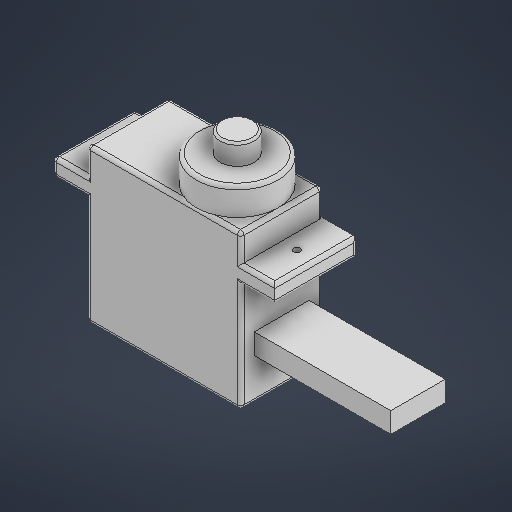
# Autodesk Inventor part: Motor
Saved by Autodesk Inventor 2026 (Build 300175000, 175)
## iProperties
Created: 2026-02-13
Part Number: Motor
Material: Generisch
Document SubType Name: Modeling
Designer: Jakob Dorninger
Density: 1 g/cm^3
Appearance: Vorgabe
Author: Jakob Dorninger
Autodesk Inventor part; units mm, degrees
ref_plane "YZ Plane" through (0, 0, 0) normal (1, 0, 0) x (0, 1, 0)
ref_plane "XZ Plane" through (0, 0, 0) normal (0, 1, 0) x (-1, 0, 0)
ref_plane "XY Plane" through (0, 0, 0) normal (0, 0, 1) x (1, 0, 0)
sketch "Skizze1" plane through (0, 0, 0) normal (0, 1, 0) x (-1, 0, 0)
  line L0 (-11.25, 0) -> (11.25, 0)
  line L1 (11.25, 0) -> (11.25, 16)
  line L2 (11.25, 16) -> (16.25, 16)
  line L3 (16.25, 16) -> (16.25, 18.5)
  line L4 (16.25, 18.5) -> (11.25, 18.5)
  line L5 (11.25, 18.5) -> (11.25, 22.5)
  line L6 (11.25, 22.5) -> (0, 22.5)
  line L7 (0, -4.5) -> (0, 27) projected
  line L8 (-11.25, 0) -> (-11.25, 16)
  line L9 (-11.25, 16) -> (-16.25, 16)
  line L10 (-16.25, 16) -> (-16.25, 18.5)
  line L11 (-16.25, 18.5) -> (-11.25, 18.5)
  line L12 (-11.25, 18.5) -> (-11.25, 22.5)
  line L13 (-11.25, 22.5) -> (0, 22.5)
  point P0 (0, 0)
  dimension "d0" = 22.5
  dimension "d1" = 16
  dimension "d2" = 5
  dimension "d3" = 2.5
  dimension "d4" = 4
  dimension "d5" = 0
  constraints: 26 end point, 5 symmetric about line, 4 perpendicular, 2 point on line, 2 vertical, 1 horizontal, 1 midpoint
  measures "d0" distance of L0.start L0.end
  measures "d1" distance of L0.end L1.end
  measures "d2" distance of L1.end L2.end
  measures "d3" distance of L2.end L3.end
  measures "d4" distance of L4.end L5.end
  measures "d5" distance from line of L6.end L7
extrude "Extrusion1" add sketch "Skizze1" along normal mid plane 12
fillet "Rundung1" radius 0.5 29 edges at (0, -6, 22.5) (11.25, 0, 0) (11.25, -6, 8) (11.25, -6, 20.5) (11.25, 6, 20.5) (-11.25, 0, 22.5) (11.25, 0, 22.5) (0, 6, 22.5) (-11.25, -6, 8) (-11.25, -6, 20.5) (-13.75, -6, 18.5) (-13.75, -6, 16) (-16.25, -6, 17.25) (13.75, -6, 18.5) (13.75, -6, 16) (16.25, 0, 16) (16.25, 0, 18.5) (16.25, 6, 17.25) (11.25, 6, 8) (-11.25, 6, 20.5) (-13.75, 6, 18.5) (-16.25, 6, 17.25) (-16.25, 0, 18.5) (-16.25, 0, 16) (-13.75, 6, 16) (-11.25, 6, 8) (-11.25, 0, 0) (0, 6, 0) (0, -6, 0)
sketch "Skizze2" plane through (-10.75, 5.5, 22.5) normal (0, 0, 1) x (1, 0, 0)
  circle A0 centre (15.5, -5.5) radius 6
  line L0 (21.5, 0) -> (21.5, -11) projected
  line L1 (21.5, 0.5) -> (0, 0.5) projected
  point P0 (10.75, -5.5)
  point P1 (21.5, -5.5)
  point P2 (21.5, -5.5)
  dimension "d9" = 6
  constraints: 2 midpoint, 1 centre point, 1 horizontal alignment, 1 tangent
  measures "d9" distance of point (21.5, -5.5) A0.centre
extrude "Extrusion2" add sketch "Skizze2" along normal blind 4
sketch "Skizze3" plane through (4.75, 0, 26.5) normal (0, 0, 1) x (1, 0, 0)
  circle A0 centre (0, 0) radius 2.5
  arc A1 (2.3979, 5.5) -> (-2.3979, 5.5) centre (0, 0) ccw projected
  point P0 (0, 6)
  point P1 (6, 0)
  dimension "d14" = 5
  constraints: 1 centre point, 1 horizontal alignment, 1 point on circle, 1 vertical alignment
  measures "d14" diameter of A0
extrude "Extrusion3" add sketch "Skizze3" along normal blind 3
fillet "Rundung2" radius 0.5 1 edges at (-1.25, 0, 26.5)
chamfer "Fasen1" distance 0.3 angle 45 1 edges at (2.25, 0, 29.5)
sketch "Skizze4" plane through (11.25, -5.5, 0.5) normal (1, 0, 0) x (0, 0, -1)
  line L0 (-8.5, 1.5) -> (-5.5, 1.5)
  line L1 (-5.5, 1.5) -> (-5.5, 9.5)
  line L2 (-5.5, 9.5) -> (-8.5, 9.5)
  line L3 (-8.5, 9.5) -> (-8.5, 1.5)
  line L4 (0.5, 0) -> (0.5, 11) projected
  point P0 (0.5, 5.5)
  point P1 (-5.5, 5.5)
  point P2 (0.5, 5.5)
  dimension "d21" = 8
  dimension "d22" = 3
  dimension "d23" = 6
  constraints: 8 end point, 2 midpoint, 2 parallel, 1 horizontal, 1 horizontal alignment, 1 perpendicular
  measures "d21" distance of L2.end L0.start
  measures "d22" distance of L1.end L2.end
  measures "d23" distance between parallel lines of L4 L1
extrude "Extrusion4" add sketch "Skizze4" along normal blind 20
sketch "Skizze5" plane through (10.75, 6, 18.5) normal (0, 0, 1) x (1, 0, 0)
  circle A0 centre (-6, -6) radius 2.2 projected
  line L0 (-26.5, -0.5) -> (-22, -0.5) projected
  point P0 (-10.75, -6)
  point P1 (2.75, -6)
  point P2 (-24.25, -6)
  point P3 (-24.25, -0.5)
  dimension "d26" = 27
  constraints: 2 horizontal alignment, 1 midpoint, 1 vertical alignment
  measures "d26" distance of point (2.75, -6) point (-24.25, -6)
hole "Bohrung1" at (13.5, 0, 18.5) at (-13.5, 0, 18.5) direction (0, 0, -1) diameter 1 depth 8 tip angle 118
